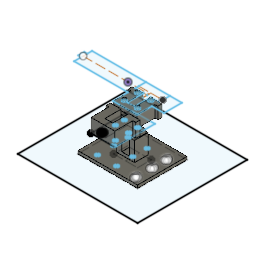
launcher v22 (Autodesk Fusion 360 design; units mm, degrees)
Autodesk Fusion 360 part; units mm, degrees
sketch "草图5" plane through (0, 0, 0) normal (0, 0, 1) x (1, 0, 0)
  line L0 (75, 15) -> (75, -15)
  line L1 (75, 15) -> (-75, 15)
  line L2 (-75, 0) -> (35, 0) construction
  line L3 (35, 3) -> (35, -3) construction
  line L4 (15, 3) -> (55, 3) construction
  line L5 (15, 3) -> (15, -3)
  line L6 (55, -3) -> (55, 3)
  line L7 (55.0002, -15) -> (55.0002, -40)
  line L8 (55.0002, -40) -> (15, -40)
  line L9 (15, -40) -> (15, -15)
  line L10 (35, -3) -> (35.0001, -3)
  line L11 (35.0001, -3) -> (35.0001, -10) construction
  line L12 (35.0001, -10) -> (35, -10)
  line L13 (35, -10) -> (35, -3) construction
  line L14 (29.0001, -3) -> (29.0001, -30)
  line L15 (40.9999, -3) -> (40.9999, -30)
  line L16 (29.0001, -30) -> (40.9999, -30)
  line L17 (55.0002, -15) -> (75, -15)
  line L18 (-75, -15) -> (15, -15)
  line L19 (35, -10) -> (35.0001, -10) construction
  line L20 (29.0001, -3) -> (35.0001, -3) construction
  line L21 (40.9999, -3) -> (42.0001, -3) construction
  line L22 (40.9999, -3) -> (55, -3)
  line L23 (15, -3) -> (29.0001, -3)
  line L24 (35, -3) -> (35.0001, -3)
  line L25 (25, -7) -> (25, -5)
  line L26 (27, -7) -> (27, -9)
  line L27 (23, -5) -> (23, -7)
  line L28 (23, -11) -> (23, -9)
  line L29 (25, -7) -> (27, -7)
  line L30 (25, -9) -> (25, -11)
  line L31 (21, -9) -> (23, -9)
  line L32 (25, -9) -> (25, -7) construction
  line L33 (25, -7) -> (25, -9) construction
  line L34 (25, -9) -> (23, -9) construction
  line L35 (23, -7) -> (21, -7)
  line L36 (23, -9) -> (23, -7) construction
  line L37 (23, -7) -> (25, -7) construction
  line L38 (23, -9) -> (25, -9) construction
  line L39 (21, -7) -> (21, -9)
  line L40 (23, -7) -> (25, -7) construction
  line L41 (27, -9) -> (25, -9)
  line L42 (25, -11) -> (23, -11)
  line L43 (23, -9) -> (23, -7) construction
  line L44 (25, -5) -> (23, -5)
  line L45 (47, -11) -> (47, -9)
  line L46 (47, -9) -> (47, -7) construction
  line L47 (45, -9) -> (47, -9) construction
  line L48 (47, -7) -> (49, -7)
  line L49 (45, -7) -> (45, -9) construction
  line L50 (43, -9) -> (45, -9)
  line L51 (47, -5) -> (47, -7)
  line L52 (45, -11) -> (47, -11)
  line L53 (49, -9) -> (47, -9)
  line L54 (47, -9) -> (45, -9) construction
  line L55 (45, -5) -> (47, -5)
  line L56 (47, -7) -> (45, -7) construction
  line L57 (45, -9) -> (45, -11)
  line L58 (45, -7) -> (43, -7)
  line L59 (47, -9) -> (47, -7) construction
  line L60 (45, -9) -> (45, -7) construction
  line L61 (45, -7) -> (45, -5)
  line L62 (49, -7) -> (49, -9)
  line L63 (43, -7) -> (43, -9)
  line L64 (47, -7) -> (45, -7) construction
  line L65 (25, -31) -> (25, -29) construction
  line L66 (27, -29) -> (27, -31)
  line L67 (25, -29) -> (27, -29)
  line L68 (23, -31) -> (23, -29) construction
  line L69 (25, -29) -> (25, -31) construction
  line L70 (25, -31) -> (25, -33)
  line L71 (21, -31) -> (23, -31)
  line L72 (23, -29) -> (25, -29) construction
  line L73 (25, -33) -> (23, -33)
  line L74 (21, -29) -> (21, -31)
  line L75 (25, -27) -> (23, -27)
  line L76 (27, -31) -> (25, -31)
  line L77 (25, -31) -> (23, -31) construction
  line L78 (23, -31) -> (25, -31) construction
  line L79 (23, -33) -> (23, -31)
  line L80 (23, -31) -> (23, -29) construction
  line L81 (23, -27) -> (23, -29)
  line L82 (23, -29) -> (25, -29) construction
  line L83 (23, -29) -> (21, -29)
  line L84 (25, -29) -> (25, -27)
  line L85 (47, -31) -> (47, -29) construction
  line L86 (49, -29) -> (49, -31)
  line L87 (43, -29) -> (43, -31)
  line L88 (47, -27) -> (47, -29)
  line L89 (45, -31) -> (45, -29) construction
  line L90 (49, -31) -> (47, -31)
  line L91 (47, -29) -> (49, -29)
  line L92 (47, -29) -> (45, -29) construction
  line L93 (45, -29) -> (45, -31) construction
  line L94 (45, -31) -> (47, -31) construction
  line L95 (45, -29) -> (45, -27)
  line L96 (45, -27) -> (47, -27)
  line L97 (45, -31) -> (45, -33)
  line L98 (47, -33) -> (47, -31)
  line L99 (47, -31) -> (45, -31) construction
  line L100 (47, -31) -> (47, -29) construction
  line L101 (45, -29) -> (43, -29)
  line L102 (47, -29) -> (45, -29) construction
  line L103 (43, -31) -> (45, -31)
  line L104 (45, -33) -> (47, -33)
  line L105 (-75, 7) -> (-75, -3) construction
  line L106 (-75, 7) -> (-80, 7)
  line L107 (-75, -3) -> (-80, -3)
  line L108 (-80, -3) -> (-80, 7)
  line L109 (-75, 15) -> (-75, 7)
  line L110 (-75, -3) -> (-75, -15)
  line L111 (15, 3) -> (15, 15)
  line L112 (55, 3) -> (55, 15)
  point P0 (55, 3)
  dimension "d46" = 30
  dimension "d47" = 110
  dimension "d48" = 150
  dimension "d49" = 6
  dimension "d50" = 40
  dimension "d51" = 13
  dimension "d52" = 27
  dimension "d60" = 2
  dimension "d61" = 2
  dimension "d62" = 2
  dimension "d63" = 2
  dimension "d64" = 2
  dimension "d65" = 2
  dimension "d66" = 2
  dimension "d67" = 2
  dimension "d68" = 2
  dimension "d69" = 2
  dimension "d70" = 2
  dimension "d71" = 2
  dimension "d148" = 10
  dimension "d149" = 5
  constraint vertical L0
  constraint perpendicular L1 L109
  constraint perpendicular L0 L1
  constraint perpendicular L2 L3
  constraint midpoint L2.end L3
  constraint horizontal L4
  constraint midpoint L3.start L4
  constraint symmetric L2 P0 L6.start
  constraint perpendicular L5 L23
  constraint vertical L7
  constraint horizontal L8
  constraint vertical L9
  constraint vertical L11
  constraint horizontal L12
  constraint vertical L13
  constraint coincident L21.end L23
  constraint parallel L20 L23
  constraint perpendicular L14 L23
  constraint symmetric L13 L14.start L15.start
  constraint symmetric L13 L14.end L15.end
  constraint collinear L17 L18
  constraint collinear L20 L21
  constraint collinear L22 L23
  constraint collinear L23 L24
  constraint horizontal L37
  constraint vertical L33
  constraint horizontal L34
  constraint vertical L36
  constraint horizontal L29
  constraint vertical L26
  constraint horizontal L41
  constraint vertical L32
  constraint horizontal L35
  constraint vertical L39
  constraint horizontal L31
  constraint vertical L43
  constraint horizontal L40
  constraint vertical L25
  constraint horizontal L44
  constraint vertical L27
  constraint horizontal L38
  constraint vertical L30
  constraint horizontal L42
  constraint vertical L28
  constraint symmetric L3 L4.start P0
  constraint symmetric L3 L35.end L48.end
  constraint symmetric L3 L31.start L53.start
  constraint symmetric L3 L26.start L58.end
  constraint symmetric L3 L25.start L49.start
  constraint symmetric L3 L27.end L46.end
  constraint symmetric L3 L25.end L55.start
  constraint symmetric L3 L27.start L51.start
  constraint symmetric L3 L30.start L47.start
  constraint symmetric L3 L30.end L52.start
  constraint symmetric L3 L28.start L45.start
  constraint symmetric L3 L28.end L45.end
  constraint symmetric L3 L26.end L50.start
  constraint horizontal L82
  constraint vertical L69
  constraint horizontal L77
  constraint vertical L68
  constraint horizontal L67
  constraint vertical L66
  constraint horizontal L76
  constraint vertical L65
  constraint horizontal L83
  constraint vertical L74
  constraint horizontal L71
  constraint vertical L80
  constraint horizontal L72
  constraint vertical L84
  constraint horizontal L75
  constraint vertical L81
  constraint horizontal L78
  constraint vertical L70
  constraint horizontal L73
  constraint vertical L79
  constraint symmetric L3 L65.start L89.start
  constraint symmetric L3 L68.start L85.start
  constraint symmetric L3 L70.end L97.end
  constraint symmetric L3 L73.end L98.start
  constraint symmetric L3 L66.end L87.end
  constraint symmetric L3 L75.start L95.end
  constraint symmetric L3 L65.end L89.end
  constraint symmetric L3 L75.end L88.start
  constraint symmetric L3 L68.end L85.end
  constraint symmetric L3 L74.start L86.start
  constraint symmetric L3 L66.start L87.start
  constraint symmetric L3 L71.start L86.end
  constraint symmetric L7 L9 L11
  constraint coincident L105.end L109
  constraint perpendicular L106 L109
  constraint perpendicular L105 L107
  constraint equal L106 L107
  constraint collinear L109 L110
  constraint coincident L1 L111.end
  constraint perpendicular L1 L111
  constraint coincident P0 L4.end
  constraint coincident L1 L112.end
  constraint perpendicular L1 L112
  measures "d46" distance of L1.end L18.start
  measures "d47" distance of L2.start L2.end
  measures "d48" distance of L1.end L0.start
  measures "d49" distance of L3.start L3.end
  measures "d50" distance of L4.start P0
  measures "d51" distance of L14.start L21.end
  measures "d52" distance of L14.start L14.end
  measures "d60" distance of L27.end L28.end
  measures "d61" distance of L27.end L25.start
  measures "d62" distance of L26.start L25.start
  measures "d63" distance of L35.end L27.end
  measures "d64" distance of L27.end L27.start
  measures "d65" distance of L28.start L28.end
  measures "d66" distance of L68.start L68.end
  measures "d67" distance of L65.end L68.end
  measures "d68" distance of L65.end L66.start
  measures "d69" distance of L68.end L74.start
  measures "d70" distance of L75.end L68.end
  measures "d71" distance of L68.start L73.end
  measures "d148" distance of L105.start L105.end
  measures "d149" distance of L105.start L106.end
sketch "草图8" plane through (0, 0, 0) normal (0, 0, 1) x (1, 0, 0)
  line L0 (49, -31) -> (47, -31)
  line L1 (43, -29) -> (43, -31)
  line L2 (45, -29) -> (43, -29)
  line L3 (45, -29) -> (45, -31) construction
  line L4 (28.5, -3) -> (28.5, -30)
  line L5 (35, -10) -> (35, -3) construction
  line L6 (27, -31) -> (25, -31)
  line L7 (27, -29) -> (27, -31)
  line L8 (23, -27) -> (23, -29)
  line L9 (25, -29) -> (27, -29)
  line L10 (41.5, -3) -> (41.5, -30)
  line L11 (43, -31) -> (45, -31)
  line L12 (25, -31) -> (25, -29) construction
  line L13 (35, -3) -> (35.0001, -3)
  line L14 (45, -33) -> (47, -33)
  line L15 (47, -31) -> (47, -29) construction
  line L16 (23, -31) -> (25, -31) construction
  line L17 (25, -33) -> (23, -33)
  line L18 (55, -10) -> (55, -40)
  line L19 (41.5, -3) -> (51, -3)
  line L20 (47, -29) -> (45, -29) construction
  line L21 (47, -29) -> (45, -29) construction
  line L22 (47, -27) -> (47, -29)
  line L23 (47, -31) -> (45, -31) construction
  line L24 (45, -27) -> (47, -27)
  line L25 (49, -29) -> (49, -31)
  line L26 (23, -31) -> (23, -29) construction
  line L27 (25, -31) -> (25, -33)
  line L28 (35, -10) -> (35.0001, -10) construction
  line L29 (35.0001, -3) -> (35.0001, -10) construction
  line L30 (35.0001, -10) -> (35, -10)
  line L31 (23, -31) -> (23, -29) construction
  line L32 (28.5, -3) -> (35.0001, -3) construction
  line L33 (23, -33) -> (23, -31)
  line L34 (23, -29) -> (25, -29) construction
  line L35 (45, -5) -> (47, -5)
  line L36 (47, -7) -> (45, -7) construction
  line L37 (45, -9) -> (45, -7) construction
  line L38 (47, -7) -> (49, -7)
  line L39 (21, -31) -> (23, -31)
  line L40 (23, -29) -> (21, -29)
  line L41 (47, -11) -> (47, -9)
  line L42 (47, -5) -> (47, -7)
  line L43 (49, -7) -> (49, -9)
  line L44 (19, -3) -> (28.5, -3)
  line L45 (45, -7) -> (45, -9) construction
  line L46 (55, -40) -> (15, -40)
  line L47 (49, -9) -> (47, -9)
  line L48 (23, -7) -> (21, -7)
  line L49 (47, -7) -> (45, -7) construction
  line L50 (28.5, -30) -> (41.5, -30)
  line L51 (45, -11) -> (47, -11)
  line L52 (21, -29) -> (21, -31)
  line L53 (25, -7) -> (25, -5)
  line L54 (45, -7) -> (43, -7)
  line L55 (43, -7) -> (43, -9)
  line L56 (15, -40) -> (15, -10)
  line L57 (47, -33) -> (47, -31)
  line L58 (45, -29) -> (45, -27)
  line L59 (45, -31) -> (45, -29) construction
  line L60 (47, -29) -> (49, -29)
  line L61 (23, -29) -> (25, -29) construction
  line L62 (25, -27) -> (23, -27)
  line L63 (25, -29) -> (25, -27)
  line L64 (25, -29) -> (25, -31) construction
  line L65 (25, -31) -> (23, -31) construction
  line L66 (35, -3) -> (35.0001, -3)
  line L67 (25, -7) -> (27, -7)
  line L68 (23, -7) -> (25, -7) construction
  line L69 (27, -7) -> (27, -9)
  line L70 (25, -7) -> (25, -9) construction
  line L71 (47, -9) -> (47, -7) construction
  line L72 (45, -9) -> (47, -9) construction
  line L73 (27, -9) -> (25, -9)
  line L74 (23, -5) -> (23, -7)
  line L75 (25, -5) -> (23, -5)
  line L76 (23, -9) -> (23, -7) construction
  line L77 (21, -9) -> (23, -9)
  line L78 (25, -9) -> (25, -11)
  line L79 (23, -9) -> (25, -9) construction
  line L80 (25, -9) -> (25, -7) construction
  line L81 (25, -11) -> (23, -11)
  line L82 (25, -9) -> (23, -9) construction
  line L83 (47, -9) -> (47, -7) construction
  line L84 (23, -7) -> (25, -7) construction
  line L85 (21, -7) -> (21, -9)
  line L86 (43, -9) -> (45, -9)
  line L87 (47, -9) -> (45, -9) construction
  line L88 (23, -9) -> (23, -7) construction
  line L89 (45, -9) -> (45, -11)
  line L90 (23, -11) -> (23, -9)
  line L91 (45, -31) -> (47, -31) construction
  line L92 (45, -31) -> (45, -33)
  line L93 (41.5, -3) -> (42.0001, -3) construction
  line L94 (47, -31) -> (47, -29) construction
  line L95 (45, -7) -> (45, -5)
  line L96 (15, -10) -> (10, -10)
  line L97 (55, -10) -> (60, -10)
  line L98 (28.5, -13.5) -> (41.5, -13.5)
  line L99 (28.5, -10.5) -> (41.5, -10.5)
  line L100 (35, -10) -> (35, -30) construction
  line L101 (10, -3) -> (60, -3)
  line L102 (10, -3) -> (10, -10)
  line L103 (60, -3) -> (60, -10)
  point P0 (35, 0)
  point P1 (51, 3)
  dimension "d90" = 27
  dimension "d91" = 2
  dimension "d92" = 2
  dimension "d93" = 2
  dimension "d94" = 2
  dimension "d95" = 2
  dimension "d96" = 2
  dimension "d97" = 2
  dimension "d98" = 2
  dimension "d99" = 2
  dimension "d100" = 2
  dimension "d101" = 2
  dimension "d102" = 2
  dimension "d105" = 16.5
  dimension "d106" = 3
  dimension "d134" = 13
  constraint vertical L18
  constraint horizontal L46
  constraint vertical L56
  constraint vertical L29
  constraint horizontal L30
  constraint vertical L5
  constraint coincident L93.end L44
  constraint parallel L32 L44
  constraint perpendicular L4 L44
  constraint symmetric L4.start L10.start L5
  constraint symmetric L10.end L4.end L5
  constraint collinear L32 L93
  constraint collinear L19 L44
  constraint collinear L13 L44
  constraint horizontal L84
  constraint vertical L70
  constraint horizontal L82
  constraint vertical L88
  constraint horizontal L67
  constraint vertical L69
  constraint horizontal L73
  constraint vertical L80
  constraint horizontal L48
  constraint vertical L85
  constraint horizontal L77
  constraint vertical L76
  constraint horizontal L68
  constraint vertical L53
  constraint horizontal L75
  constraint vertical L74
  constraint horizontal L79
  constraint vertical L78
  constraint horizontal L81
  constraint vertical L90
  constraint horizontal L61
  constraint vertical L64
  constraint horizontal L65
  constraint vertical L31
  constraint horizontal L9
  constraint vertical L7
  constraint horizontal L6
  constraint vertical L12
  constraint horizontal L40
  constraint vertical L52
  constraint horizontal L39
  constraint vertical L26
  constraint horizontal L34
  constraint vertical L63
  constraint horizontal L62
  constraint vertical L8
  constraint horizontal L16
  constraint vertical L27
  constraint horizontal L17
  constraint vertical L33
  constraint perpendicular L56 L96
  constraint coincident L4 L98.start
  constraint coincident L10 L98.end
  constraint perpendicular L10 L98
  constraint coincident L4 L99.start
  constraint coincident L10 L99.end
  constraint perpendicular L10 L99
  constraint midpoint L50 L100.end
  constraint perpendicular L96 L102
  constraint perpendicular L97 L103
  measures "d90" distance of L4.start L4.end
  measures "d91" distance of L76.start L48.start
  measures "d92" distance of L53.start L48.start
  measures "d93" distance of L53.start L67.end
  measures "d94" distance of L48.start L48.end
  measures "d95" distance of L74.start L48.start
  measures "d96" distance of L76.start L81.end
  measures "d97" distance of L8.end L16.start
  measures "d98" distance of L8.end L9.start
  measures "d99" distance of L9.start L7.start
  measures "d100" distance of L40.end L8.end
  measures "d101" distance of L8.start L8.end
  measures "d102" distance of L17.end L16.start
  measures "d105" distance of L50 L98
  measures "d106" distance of L98 L99
  measures "d134" distance of L10.end L4.end
extrude "拉伸10" add sketch "草图8" along normal blind 3 contours L0 L1 L2 L11 L14 L22 L24 L25 L57 L58 L60 L92 | L6 L7 L8 L9 L17 L27 L33 L39 L40 L52 L62 L63 | L35 L38 L41 L42 L43 L47 L51 L54 L55 L86 L89 L95 | L48 L53 L67 L69 L73 L74 L75 L77 L78 L81 L85 L90 makes body 1 at (44.3333, -8.3333, 0) makes body 2 at (46.3333, -31.6667, 0) makes body 3 at (24.3333, -9.6667, 0) makes body 4 at (22.3333, -30.3333, 0)
extrude "拉伸11" add sketch "草图8" against normal blind 20 contours L0 L1 L2 L11 L14 L22 L24 L25 L57 L58 L60 L92 | L4 L10 L99 L101 | L4 L10 L18 L19 L44 L46 L50 L56 L96 L97 L101 L102 L103 | L4 L10 L98 L99 | L4 L10 L50 L98 | L6 L7 L8 L9 L17 L27 L33 L39 L40 L52 L62 L63 | L35 L38 L41 L42 L43 L47 L51 L54 L55 L86 L89 L95 | L48 L53 L67 L69 L73 L74 L75 L77 L78 L81 L85 L90 bodies 1 2 3 4
extrude "拉伸12" cut sketch "草图8" against normal blind 17 contours L4 L10 L98 L99 | L4 L10 L50 L98 bodies 1
extrude "拉伸13" cut sketch "草图8" against normal blind 20 contours L4 L10 L98 L99 bodies 1
extrude "拉伸19" cut sketch "草图8" against normal blind 20 contours L0 L1 L2 L11 L14 L22 L24 L25 L57 L58 L60 L92 | L4 L10 L99 L101 | L4 L10 L18 L19 L44 L46 L50 L56 L96 L97 L101 L102 L103 | L4 L10 L98 L99 | L4 L10 L50 L98 | L6 L7 L8 L9 L17 L27 L33 L39 L40 L52 L62 L63 | L35 L38 L41 L42 L43 L47 L51 L54 L55 L86 L89 L95 | L48 L53 L67 L69 L73 L74 L75 L77 L78 L81 L85 L90 bodies 1 makes body 5 at (22.3333, -30.3333, 0) makes body 6 at (24.3333, -9.6667, 3) makes body 7 at (46.3333, -31.6667, 0)
sketch "草图11" plane through (0, 0, 0) normal (0, 0, 1) x (1, 0, 0)
  line L0 (15, -35, -5) -> (55, -35, -5)
  line L1 (55, -35, -5) -> (55, -35, -15)
  line L2 (55, -35, -15) -> (15, -35, -15)
  line L3 (15, -35, -15) -> (15, -35, -5)
  circle A0 through (38.5, -35, -10) (33.25, -35, -6.9689) (33.25, -35, -13.0311)
  circle A1 through (38, -35, -10) (33.5, -35, -7.4019) (33.5, -35, -12.5981) construction
  line L4 (35, -35, -5) -> (35, -35, -15) construction
  line L5 (35, -35, -10) -> (49, -35, -10) construction
  circle A2 through (51, -35, -10) (48, -35, -8.2679) (48, -35, -11.7321)
  line L6 (35, -35, -6.9923) -> (49.1429, -35, -8.0051)
  line L7 (35, -35, -13.0077) -> (49.1429, -35, -11.9949)
  line L8 (35, -35, -6.9923) -> (20.8571, -35, -8.0051)
  line L9 (35, -35, -13.0077) -> (20.8571, -35, -11.9949)
  line L10 (35, -35, -10) -> (21, -35, -10) construction
  circle A3 through (23, -35, -10) (20, -35, -8.2679) (20, -35, -11.7321)
  dimension "d141" = 7
  dimension "d142" = 6
  dimension "d143" = 4
  dimension "d154" = 14
extrude "拉伸21" add sketch "草图8" against normal blind 20 contours L0 L1 L2 L11 L14 L22 L24 L25 L57 L58 L60 L92 | L4 L10 L99 L101 | L4 L10 L18 L19 L44 L46 L50 L56 L96 L97 L101 L102 L103 | L4 L10 L50 L98 | L6 L7 L8 L9 L17 L27 L33 L39 L40 L52 L62 L63 | L35 L38 L41 L42 L43 L47 L51 L54 L55 L86 L89 L95 | L48 L53 L67 L69 L73 L74 L75 L77 L78 L81 L85 L90 bodies 1 5 6 7
extrude "拉伸22" cut sketch "草图8" against normal blind 17 contours L4 L10 L99 L101 | L4 L10 L50 L98 bodies 1
extrude "拉伸23" cut sketch "草图11" against normal blind 6 contours A0 L6 L7 L8 L9 | A0 L8 L9 A3 | A0 L6 L8 | A0 L7 L9 | A0 A2 L6 L7 | A3 | A2 in plane through (0, -35, 0) normal (0, 1, 0) bodies 1
copy_body "复制和粘贴实体1" bodies 1 makes body 8
move_body "移动1" bodies 8 to x (1, 0, 0) y (0, 1, 0) z (0, 0, 1) at (-72, -41, 20)
extrude "拉伸24" add 1 faces at (-43.0559, -76, 9.335) along direction (0, -1, 0) blind 5 on bodies 8 bodies 8
extrude "拉伸25" add 4 faces at (-27.6667, -49.3333, 23) (-49.6667, -48.6667, 23) (-49.6667, -71.3333, 23) (-25.6667, -72.6667, 23) along direction (0, 0, -1) blind 28 on bodies 8 bodies 8
extrude "拉伸26" cut 4 faces at (-49.6667, -48.6667, 23) (-27.6667, -49.3333, 23) (-25.6667, -72.6667, 23) (-49.6667, -71.3333, 23) along direction (0, 0, -1) blind 3 on bodies 8 bodies 8
extrude "拉伸27" add 1 faces at (-39.1667, -64.8333, 0) along direction (0, 0, -1) blind 2 on bodies 8 bodies 8
extrude "拉伸28" add 1 faces at (-39.1667, -64.8333, -2) along direction (0, 0, -1) blind 1 on bodies 8 bodies 8
extrude "拉伸29" add 4 faces at (-27.6667, -49.3333, -5) (-49.6667, -48.6667, -5) (-49.6667, -71.3333, -5) (-25.6667, -72.6667, -5) along direction (0, 0, -1) blind 1 on bodies 8 bodies 8
move_body "移动2" bodies 8 to x (1, 0, 0) y (0, 1, 0) z (0, 0, 1) at (72, 4, -25)
sketch "草图12" plane through (0, 0, -28) normal (0, 0, -1) x (1, 0, 0)
  line L0 (43, 66) -> (43, 68)
  line L1 (43, 68) -> (45, 68)
  line L2 (45, 68) -> (45, 70)
  line L3 (45, 70) -> (47, 70)
  line L4 (47, 70) -> (47, 68)
  line L5 (47, 68) -> (49, 68)
  line L6 (49, 68) -> (49, 66)
  line L7 (49, 66) -> (47, 66)
  line L8 (47, 66) -> (47, 64)
  line L9 (47, 64) -> (45, 64)
  line L10 (45, 64) -> (45, 66)
  line L11 (45, 66) -> (43, 66)
  line L12 (25, 42) -> (23, 42)
  line L13 (23, 42) -> (23, 44)
  line L14 (23, 44) -> (21, 44)
  line L15 (21, 44) -> (21, 46)
  line L16 (21, 46) -> (23, 46)
  line L17 (23, 46) -> (23, 48)
  line L18 (23, 48) -> (25, 48)
  line L19 (25, 48) -> (25, 46)
  line L20 (25, 46) -> (27, 46)
  line L21 (27, 46) -> (27, 44)
  line L22 (27, 44) -> (25, 44)
  line L23 (25, 44) -> (25, 42)
  line L24 (43, 46) -> (45, 46)
  line L25 (45, 46) -> (45, 48)
  line L26 (45, 48) -> (47, 48)
  line L27 (47, 48) -> (47, 46)
  line L28 (47, 46) -> (49, 46)
  line L29 (49, 46) -> (49, 44)
  line L30 (49, 44) -> (47, 44)
  line L31 (47, 44) -> (47, 42)
  line L32 (47, 42) -> (45, 42)
  line L33 (45, 42) -> (45, 44)
  line L34 (45, 44) -> (43, 44)
  line L35 (43, 44) -> (43, 46)
  line L36 (25, 66) -> (25, 64)
  line L37 (25, 64) -> (23, 64)
  line L38 (23, 64) -> (23, 66)
  line L39 (23, 66) -> (21, 66)
  line L40 (21, 66) -> (21, 68)
  line L41 (21, 68) -> (23, 68)
  line L42 (23, 68) -> (23, 70)
  line L43 (23, 70) -> (25, 70)
  line L44 (25, 70) -> (25, 68)
  line L45 (25, 68) -> (27, 68)
  line L46 (27, 68) -> (27, 66)
  line L47 (27, 66) -> (25, 66)
  line L48 (28.5, 50.5) -> (41.5, 50.5)
  line L49 (41.5, 50.5) -> (41.5, 47.5)
  line L50 (41.5, 47.5) -> (28.5, 47.5)
  line L51 (28.5, 47.5) -> (28.5, 50.5)
  line L52 (10, 47) -> (10, 40)
  line L53 (10, 40) -> (60, 40)
  line L54 (60, 40) -> (60, 47)
  line L55 (60, 47) -> (55, 47)
  line L56 (55, 47) -> (55, 77)
  line L57 (55, 77) -> (15, 77)
  line L58 (15, 77) -> (15, 47)
  line L59 (15, 47) -> (10, 47)
  line L60 (15, 77) -> (55, 77)
  line L61 (55, 77) -> (55, 10)
  line L62 (55, 10) -> (15, 10)
  line L63 (15, 10) -> (15, 77)
  line L64 (21, 68) -> (23, 68)
  line L65 (23, 70) -> (25, 70)
  line L66 (25, 68) -> (27, 68)
  line L67 (27, 66) -> (25, 66)
  line L68 (25, 64) -> (23, 64)
  line L69 (23, 66) -> (21, 66)
  line L70 (25, 70) -> (25, 68)
  line L71 (27, 68) -> (27, 66)
  line L72 (25, 66) -> (25, 64)
  line L73 (23, 64) -> (23, 66)
  line L74 (21, 66) -> (21, 68)
  line L75 (23, 68) -> (23, 70)
  line L76 (47, 66) -> (47, 64)
  line L77 (49, 66) -> (47, 66)
  line L78 (45, 66) -> (43, 66)
  line L79 (43, 68) -> (45, 68)
  line L80 (43, 66) -> (43, 68)
  line L81 (45, 64) -> (45, 66)
  line L82 (47, 64) -> (45, 64)
  line L83 (47, 70) -> (47, 68)
  line L84 (47, 64) -> (45, 64)
  line L85 (47, 70) -> (47, 68)
  line L86 (49, 68) -> (49, 66)
  line L87 (47, 68) -> (49, 68)
  line L88 (45, 68) -> (45, 70)
  line L89 (43, 66) -> (43, 68)
  line L90 (47, 66) -> (47, 64)
  line L91 (45, 64) -> (45, 66)
  line L92 (43, 68) -> (45, 68)
  line L93 (49, 66) -> (47, 66)
  line L94 (45, 70) -> (47, 70)
  line L95 (47, 68) -> (49, 68)
  line L96 (45, 68) -> (45, 70)
  line L97 (45, 66) -> (43, 66)
  line L98 (45, 70) -> (47, 70)
  line L99 (49, 68) -> (49, 66)
  line L100 (47, 46) -> (49, 46)
  line L101 (49, 46) -> (49, 44)
  line L102 (49, 44) -> (47, 44)
  line L103 (47, 44) -> (47, 42)
  line L104 (25, 46) -> (27, 46)
  line L105 (45, 42) -> (45, 44)
  line L106 (27, 46) -> (27, 44)
  line L107 (25, 46) -> (27, 46)
  line L108 (23, 48) -> (25, 48)
  line L109 (45, 44) -> (43, 44)
  line L110 (27, 44) -> (25, 44)
  line L111 (45, 48) -> (47, 48)
  line L112 (45, 46) -> (45, 48)
  line L113 (47, 44) -> (47, 42)
  line L114 (47, 44) -> (47, 42)
  line L115 (21, 46) -> (23, 46)
  line L116 (49, 44) -> (47, 44)
  line L117 (25, 48) -> (25, 46)
  line L118 (49, 46) -> (49, 44)
  line L119 (45, 42) -> (45, 44)
  line L120 (25, 44) -> (25, 42)
  line L121 (21, 44) -> (21, 46)
  line L122 (23, 46) -> (23, 48)
  line L123 (27, 46) -> (27, 44)
  line L124 (23, 42) -> (23, 44)
  line L125 (21, 46) -> (23, 46)
  line L126 (49, 44) -> (47, 44)
  line L127 (25, 42) -> (23, 42)
  line L128 (23, 44) -> (21, 44)
  line L129 (23, 48) -> (25, 48)
  line L130 (23, 42) -> (23, 44)
  line L131 (23, 46) -> (23, 48)
  line L132 (25, 42) -> (23, 42)
  line L133 (23, 44) -> (21, 44)
  line L134 (25, 44) -> (25, 42)
  line L135 (47, 42) -> (45, 42)
  line L136 (45, 46) -> (45, 48)
  line L137 (47, 48) -> (47, 46)
  line L138 (25, 48) -> (25, 46)
  line L139 (21, 44) -> (21, 46)
  line L140 (45, 48) -> (47, 48)
  line L141 (43, 46) -> (45, 46)
  line L142 (49, 46) -> (49, 44)
  line L143 (27, 44) -> (25, 44)
  line L144 (43, 44) -> (43, 46)
  line L145 (47, 48) -> (47, 46)
  line L146 (47, 46) -> (49, 46)
  line L147 (47, 48) -> (47, 46)
  line L148 (45, 46) -> (45, 48)
  line L149 (45, 48) -> (47, 48)
  line L150 (47, 46) -> (49, 46)
  line L151 (47, 42) -> (45, 42)
  line L152 (45, 44) -> (43, 44)
  line L153 (43, 46) -> (45, 46)
  line L154 (43, 44) -> (43, 46)
  line L155 (43, 44) -> (43, 46)
  line L156 (45, 42) -> (45, 44)
  line L157 (45, 44) -> (43, 44)
  line L158 (47, 42) -> (45, 42)
  line L159 (43, 46) -> (45, 46)
  line L160 (47, 31) -> (49, 31)
  line L161 (49, 31) -> (49, 29)
  line L162 (49, 29) -> (47, 29)
  line L163 (47, 29) -> (47, 27)
  line L164 (25, 31) -> (27, 31)
  line L165 (45, 27) -> (45, 29)
  line L166 (27, 31) -> (27, 29)
  line L167 (25, 31) -> (27, 31)
  line L168 (23, 33) -> (25, 33)
  line L169 (45, 29) -> (43, 29)
  line L170 (27, 29) -> (25, 29)
  line L171 (45, 33) -> (47, 33)
  line L172 (45, 31) -> (45, 33)
  line L173 (47, 29) -> (47, 27)
  line L174 (47, 29) -> (47, 27)
  line L175 (21, 31) -> (23, 31)
  line L176 (49, 29) -> (47, 29)
  line L177 (25, 33) -> (25, 31)
  line L178 (49, 31) -> (49, 29)
  line L179 (45, 27) -> (45, 29)
  line L180 (25, 29) -> (25, 27)
  line L181 (21, 29) -> (21, 31)
  line L182 (23, 31) -> (23, 33)
  line L183 (27, 31) -> (27, 29)
  line L184 (23, 27) -> (23, 29)
  line L185 (21, 31) -> (23, 31)
  line L186 (49, 29) -> (47, 29)
  line L187 (25, 27) -> (23, 27)
  line L188 (23, 29) -> (21, 29)
  line L189 (23, 33) -> (25, 33)
  line L190 (23, 27) -> (23, 29)
  line L191 (23, 31) -> (23, 33)
  line L192 (25, 27) -> (23, 27)
  line L193 (23, 29) -> (21, 29)
  line L194 (25, 29) -> (25, 27)
  line L195 (47, 27) -> (45, 27)
  line L196 (45, 31) -> (45, 33)
  line L197 (47, 33) -> (47, 31)
  line L198 (25, 33) -> (25, 31)
  line L199 (21, 29) -> (21, 31)
  line L200 (45, 33) -> (47, 33)
  line L201 (43, 31) -> (45, 31)
  line L202 (49, 31) -> (49, 29)
  line L203 (27, 29) -> (25, 29)
  line L204 (43, 29) -> (43, 31)
  line L205 (47, 33) -> (47, 31)
  line L206 (47, 31) -> (49, 31)
  line L207 (47, 33) -> (47, 31)
  line L208 (45, 31) -> (45, 33)
  line L209 (45, 33) -> (47, 33)
  line L210 (47, 31) -> (49, 31)
  line L211 (47, 27) -> (45, 27)
  line L212 (45, 29) -> (43, 29)
  line L213 (43, 31) -> (45, 31)
  line L214 (43, 29) -> (43, 31)
  line L215 (43, 29) -> (43, 31)
  line L216 (45, 27) -> (45, 29)
  line L217 (45, 29) -> (43, 29)
  line L218 (47, 27) -> (45, 27)
  line L219 (43, 31) -> (45, 31)
  constraint horizontal L60
  constraint vertical L61
  constraint horizontal L62
  constraint vertical L63
  constraint coincident L57.end L58.start
  constraint coincident L40.end L41.start
  constraint coincident L41.end L42.start
  constraint coincident L42.end L43.start
  constraint coincident L43.end L44.start
  constraint coincident L44.end L45.start
  constraint coincident L45.end L46.start
  constraint coincident L46.end L47.start
  constraint coincident L36.start L47.end
  constraint coincident L36.end L37.start
  constraint coincident L37.end L38.start
  constraint coincident L38.end L39.start
  constraint coincident L39.end L40.start
  constraint coincident L0.end L1.start
  constraint coincident L1.end L2.start
  constraint coincident L2.end L3.start
  constraint coincident L3.end L4.start
  constraint coincident L4.end L5.start
  constraint coincident L5.end L6.start
  constraint coincident L6.end L7.start
  constraint coincident L7.end L8.start
  constraint coincident L8.end L9.start
  constraint coincident L9.end L10.start
  constraint coincident L10.end L11.start
  constraint coincident L0.start L11.end
  constraint coincident L15.end L16.start
  constraint coincident L16.end L17.start
  constraint coincident L17.end L18.start
  constraint coincident L18.end L19.start
  constraint coincident L19.end L20.start
  constraint coincident L20.end L21.start
  constraint coincident L21.end L22.start
  constraint coincident L22.end L23.start
  constraint coincident L12.start L23.end
  constraint coincident L12.end L13.start
  constraint coincident L13.end L14.start
  constraint coincident L14.end L15.start
  constraint coincident L24.start L35.end
  constraint coincident L24.end L25.start
  constraint coincident L25.end L26.start
  constraint coincident L26.end L27.start
  constraint coincident L27.end L28.start
  constraint coincident L28.end L29.start
  constraint coincident L29.end L30.start
  constraint coincident L30.end L31.start
  constraint coincident L31.end L32.start
  constraint coincident L32.end L33.start
  constraint coincident L33.end L34.start
  constraint coincident L34.end L35.start
  constraint coincident L175.start L181.end
  constraint coincident L175.end L182.start
  constraint coincident L168.start L182.end
  constraint coincident L168.end L177.start
  constraint coincident L164.start L167.start
  constraint coincident L164.end L166.start
  constraint coincident L166.end L170.start
  constraint coincident L170.end L180.start
  constraint coincident L180.end L187.start
  constraint coincident L184.start L187.end
  constraint coincident L184.end L188.start
  constraint coincident L181.start L188.end
  constraint coincident L201.start L204.end
  constraint coincident L172.start L196.start
  constraint coincident L171.start L172.end
  constraint coincident L171.end L197.start
  constraint coincident L160.start L197.end
  constraint coincident L160.end L161.start
  constraint coincident L161.end L162.start
  constraint coincident L162.end L163.start
  constraint coincident L163.end L173.end
  constraint coincident L165.start L179.start
  constraint coincident L165.end L169.start
  constraint coincident L169.end L204.start
sketch "草图13" plane through (0, 0, 0) normal (0, 1, 0) x (1, 0, 0)
  circle A0 through (19, 31, -30) (22, 31, -28.2679) (22, 31, -31.7321)
  line L0 (35, 31, -30) -> (21, 31, -30) construction
  line L1 (35, 31, -30) -> (49, 31, -30) construction
  line L2 (35, 31, -35) -> (35, 31, -25) construction
  line L3 (35, 31, -26.9923) -> (20.8571, 31, -28.0051)
  line L4 (35, 31, -33.0077) -> (20.8571, 31, -31.9949)
  line L5 (35, 31, -26.9923) -> (49.1429, 31, -28.0051)
  circle A1 through (32, 31, -30) (36.5, 31, -27.4019) (36.5, 31, -32.5981) construction
  circle A2 through (31.5, 31, -30) (36.75, 31, -26.9689) (36.75, 31, -33.0311)
  line L6 (35, 31, -33.0077) -> (49.1429, 31, -31.9949)
  line L7 (15, 31, -25) -> (15, 31, -35)
  line L8 (15, 31, -35) -> (55, 31, -35)
  line L9 (55, 31, -35) -> (55, 31, -25)
  circle A3 through (47, 31, -30) (50, 31, -28.2679) (50, 31, -31.7321)
  line L10 (55, 31, -25) -> (15, 31, -25)
  dimension "d183" = 7
  dimension "d184" = 6
  dimension "d185" = 4
  dimension "d186" = 14
extrude "拉伸35" add sketch "草图13" along normal blind 5 separate body contours A0 | A0 L3 L4 A2 | L3 L4 L5 A2 L6 | L3 L5 A2 | L4 A2 L6 | L5 A2 L6 A3 | A3 | L7 L8 L9 L10 in plane through (0, 0, -31) normal (0, 0, -1) makes body 9
extrude "拉伸36" add sketch "草图12" along normal blind 3 contours L160 L161 L162 L163 L165 L169 L171 L172 L173 L174 L176 L178 L179 L186 L195 L196 L197 L200 L201 L202 L204 L205 L206 L207 L208 L209 L210 L211 L212 L213 L214 L215 L216 L217 L218 L219 | L164 L166 L167 L168 L170 L175 L177 L180 L181 L182 L183 L184 L185 L187 L188 L189 L190 L191 L192 L193 L194 L198 L199 L203 bodies 9
extrude "拉伸37" add sketch "草图13" along normal blind 8 contours L7 L8 L9 L10 in plane through (0, 0, -31) normal (0, 0, -1) bodies 9
extrude "拉伸38" cut 1 faces at (41.0559, -29.335, -36) along direction (0, 0, 1) blind 2 on bodies 9 bodies 9
extrude "拉伸39" cut 1 faces at (16.3333, -30, -39) along direction (0, 0, 1) blind 2 on bodies 9 bodies 9
copy_body "复制和粘贴实体2" bodies 8 makes body 10
move_body "移动3" bodies 10 to x (1, 0, 0) y (0, 0, 1) z (0, -1, 0) at (0, -44, 0)
extrude "拉伸40" cut 4 faces at (22.3333, -13, -44.6667) (44.3333, -13, -45.3333) (22.3333, -13, -67.3333) (46.3333, -13, -68.6667) along direction (0, -1, 0) blind 3 on bodies 10 bodies 10
sketch "草图14" plane through (0, 0, -77) normal (0, 0, -1) x (1, 0, 0)
  line L0 (55, 39) -> (15, 39)
  line L1 (15, 39) -> (15, 16)
  line L2 (15, 16) -> (55, 16)
  line L3 (55, 16) -> (55, 39)
  line L4 (2, 57) -> (4, 57)
  line L5 (4, 57) -> (4, 55)
  line L6 (0, 55) -> (2, 55)
  line L7 (4, 57) -> (4, 55)
  line L8 (2, 55) -> (2, 57)
  line L9 (4, 55) -> (6, 55)
  line L10 (0, 55) -> (2, 55)
  line L11 (4, 55) -> (6, 55)
  line L12 (2, 57) -> (4, 57)
  line L13 (2, 55) -> (2, 57)
  line L14 (2, 53) -> (0, 53)
  line L15 (4, 53) -> (4, 51)
  line L16 (2, 53) -> (0, 53)
  line L17 (4, 51) -> (2, 51)
  line L18 (2, 51) -> (2, 53)
  line L19 (4, 51) -> (2, 51)
  line L20 (4, 53) -> (4, 51)
  line L21 (0, 53) -> (0, 55)
  line L22 (6, 55) -> (6, 53)
  line L23 (6, 55) -> (6, 53)
  line L24 (6, 53) -> (4, 53)
  line L25 (0, 53) -> (0, 55)
  line L26 (2, 51) -> (2, 53)
  line L27 (6, 53) -> (4, 53)
  line L28 (15, 39) -> (55, 39)
  line L29 (55, 39) -> (55, 16)
  line L30 (55, 16) -> (15, 16)
  line L31 (15, 16) -> (15, 39)
  line L32 (85, -14) -> (-15, -14)
  line L33 (-15, -14) -> (-15, 69)
  line L34 (-15, 69) -> (85, 69)
  line L35 (85, 69) -> (85, -14)
  line L36 (35, 39) -> (35, 16) construction
  line L37 (66, 57) -> (66, 55)
  line L38 (70, 53) -> (70, 55)
  line L39 (66, 53) -> (66, 51)
  line L40 (68, 53) -> (70, 53)
  line L41 (64, 55) -> (64, 53)
  line L42 (64, 53) -> (66, 53)
  line L43 (68, 51) -> (68, 53)
  line L44 (70, 55) -> (68, 55)
  line L45 (66, 55) -> (64, 55)
  line L46 (66, 51) -> (68, 51)
  line L47 (68, 55) -> (68, 57)
  line L48 (66, 55) -> (64, 55)
  line L49 (68, 57) -> (66, 57)
  line L50 (70, 55) -> (68, 55)
  line L51 (66, 53) -> (66, 51)
  line L52 (66, 51) -> (68, 51)
  line L53 (68, 53) -> (70, 53)
  line L54 (64, 53) -> (66, 53)
  line L55 (64, 55) -> (64, 53)
  line L56 (70, 53) -> (70, 55)
  line L57 (68, 51) -> (68, 53)
  line L58 (66, 57) -> (66, 55)
  line L59 (68, 55) -> (68, 57)
  line L60 (68, 57) -> (66, 57)
  line L61 (32, 53) -> (32, 55)
  line L62 (36, 51) -> (34, 51)
  line L63 (36, 57) -> (36, 55)
  line L64 (36, 53) -> (36, 51)
  line L65 (34, 57) -> (36, 57)
  line L66 (34, 51) -> (34, 53)
  line L67 (38, 53) -> (36, 53)
  line L68 (36, 51) -> (34, 51)
  line L69 (36, 53) -> (36, 51)
  line L70 (36, 55) -> (38, 55)
  line L71 (36, 55) -> (38, 55)
  line L72 (38, 55) -> (38, 53)
  line L73 (36, 57) -> (36, 55)
  line L74 (32, 53) -> (32, 55)
  line L75 (34, 53) -> (32, 53)
  line L76 (34, 55) -> (34, 57)
  line L77 (34, 53) -> (32, 53)
  line L78 (38, 53) -> (36, 53)
  line L79 (38, 55) -> (38, 53)
  line L80 (32, 55) -> (34, 55)
  line L81 (34, 51) -> (34, 53)
  line L82 (34, 57) -> (36, 57)
  line L83 (32, 55) -> (34, 55)
  line L84 (34, 55) -> (34, 57)
  line L85 (4, 30) -> (4, 28)
  line L86 (34, 30) -> (36, 30)
  line L87 (34, 28) -> (34, 30)
  line L88 (6, 28) -> (6, 26)
  line L89 (6, 28) -> (6, 26)
  line L90 (38, 26) -> (36, 26)
  line L91 (38, 26) -> (36, 26)
  line L92 (4, 26) -> (4, 24)
  line L93 (68, 26) -> (70, 26)
  line L94 (66, 28) -> (64, 28)
  line L95 (2, 24) -> (2, 26)
  line L96 (4, 26) -> (4, 24)
  line L97 (70, 28) -> (68, 28)
  line L98 (66, 28) -> (64, 28)
  line L99 (2, 24) -> (2, 26)
  line L100 (2, 26) -> (0, 26)
  line L101 (38, 28) -> (38, 26)
  line L102 (34, 28) -> (34, 30)
  line L103 (36, 30) -> (36, 28)
  line L104 (36, 26) -> (36, 24)
  line L105 (32, 28) -> (34, 28)
  line L106 (34, 24) -> (34, 26)
  line L107 (38, 28) -> (38, 26)
  line L108 (36, 24) -> (34, 24)
  line L109 (32, 28) -> (34, 28)
  line L110 (66, 30) -> (66, 28)
  line L111 (68, 28) -> (68, 30)
  line L112 (68, 28) -> (68, 30)
  line L113 (32, 26) -> (32, 28)
  line L114 (34, 24) -> (34, 26)
  line L115 (34, 30) -> (36, 30)
  line L116 (36, 28) -> (38, 28)
  line L117 (34, 26) -> (32, 26)
  line L118 (66, 26) -> (66, 24)
  line L119 (4, 28) -> (6, 28)
  line L120 (66, 24) -> (68, 24)
  line L121 (64, 28) -> (64, 26)
  line L122 (70, 26) -> (70, 28)
  line L123 (4, 28) -> (6, 28)
  line L124 (2, 30) -> (4, 30)
  line L125 (66, 26) -> (66, 24)
  line L126 (2, 30) -> (4, 30)
  line L127 (70, 26) -> (70, 28)
  line L128 (68, 30) -> (66, 30)
  line L129 (68, 30) -> (66, 30)
  line L130 (6, 26) -> (4, 26)
  line L131 (4, 24) -> (2, 24)
  line L132 (6, 26) -> (4, 26)
  line L133 (66, 30) -> (66, 28)
  line L134 (4, 24) -> (2, 24)
  line L135 (36, 30) -> (36, 28)
  line L136 (36, 26) -> (36, 24)
  line L137 (32, 26) -> (32, 28)
  line L138 (34, 26) -> (32, 26)
  line L139 (36, 24) -> (34, 24)
  line L140 (36, 28) -> (38, 28)
  line L141 (4, 30) -> (4, 28)
  line L142 (68, 26) -> (70, 26)
  line L143 (64, 26) -> (66, 26)
  line L144 (64, 26) -> (66, 26)
  line L145 (0, 28) -> (2, 28)
  line L146 (2, 28) -> (2, 30)
  line L147 (0, 28) -> (2, 28)
  line L148 (0, 26) -> (0, 28)
  line L149 (70, 28) -> (68, 28)
  line L150 (66, 24) -> (68, 24)
  line L151 (68, 24) -> (68, 26)
  line L152 (64, 28) -> (64, 26)
  line L153 (2, 26) -> (0, 26)
  line L154 (2, 28) -> (2, 30)
  line L155 (0, 26) -> (0, 28)
  line L156 (68, 24) -> (68, 26)
  line L157 (4, 6) -> (4, 4)
  line L158 (34, 6) -> (36, 6)
  line L159 (34, 4) -> (34, 6)
  line L160 (6, 4) -> (6, 2)
  line L161 (6, 4) -> (6, 2)
  line L162 (38, 2) -> (36, 2)
  line L163 (38, 2) -> (36, 2)
  line L164 (4, 2) -> (4, 0)
  line L165 (68, 2) -> (70, 2)
  line L166 (66, 4) -> (64, 4)
  line L167 (2, 0) -> (2, 2)
  line L168 (4, 2) -> (4, 0)
  line L169 (70, 4) -> (68, 4)
  line L170 (66, 4) -> (64, 4)
  line L171 (2, 0) -> (2, 2)
  line L172 (2, 2) -> (0, 2)
  line L173 (38, 4) -> (38, 2)
  line L174 (34, 4) -> (34, 6)
  line L175 (36, 6) -> (36, 4)
  line L176 (36, 2) -> (36, 0)
  line L177 (32, 4) -> (34, 4)
  line L178 (34, 0) -> (34, 2)
  line L179 (38, 4) -> (38, 2)
  line L180 (36, 0) -> (34, 0)
  line L181 (32, 4) -> (34, 4)
  line L182 (66, 6) -> (66, 4)
  line L183 (68, 4) -> (68, 6)
  line L184 (68, 4) -> (68, 6)
  line L185 (32, 2) -> (32, 4)
  line L186 (34, 0) -> (34, 2)
  line L187 (34, 6) -> (36, 6)
  line L188 (36, 4) -> (38, 4)
  line L189 (34, 2) -> (32, 2)
  line L190 (66, 2) -> (66, 0)
  line L191 (4, 4) -> (6, 4)
  line L192 (66, 0) -> (68, 0)
  line L193 (64, 4) -> (64, 2)
  line L194 (70, 2) -> (70, 4)
  line L195 (4, 4) -> (6, 4)
  line L196 (2, 6) -> (4, 6)
  line L197 (66, 2) -> (66, 0)
  line L198 (2, 6) -> (4, 6)
  line L199 (70, 2) -> (70, 4)
  line L200 (68, 6) -> (66, 6)
  line L201 (68, 6) -> (66, 6)
  line L202 (6, 2) -> (4, 2)
  line L203 (4, 0) -> (2, 0)
  line L204 (6, 2) -> (4, 2)
  line L205 (66, 6) -> (66, 4)
  line L206 (4, 0) -> (2, 0)
  line L207 (36, 6) -> (36, 4)
  line L208 (36, 2) -> (36, 0)
  line L209 (32, 2) -> (32, 4)
  line L210 (34, 2) -> (32, 2)
  line L211 (36, 0) -> (34, 0)
  line L212 (36, 4) -> (38, 4)
  line L213 (4, 6) -> (4, 4)
  line L214 (68, 2) -> (70, 2)
  line L215 (64, 2) -> (66, 2)
  line L216 (64, 2) -> (66, 2)
  line L217 (0, 4) -> (2, 4)
  line L218 (2, 4) -> (2, 6)
  line L219 (0, 4) -> (2, 4)
  line L220 (0, 2) -> (0, 4)
  line L221 (70, 4) -> (68, 4)
  line L222 (66, 0) -> (68, 0)
  line L223 (68, 0) -> (68, 2)
  line L224 (64, 4) -> (64, 2)
  line L225 (2, 2) -> (0, 2)
  line L226 (2, 4) -> (2, 6)
  line L227 (0, 2) -> (0, 4)
  line L228 (68, 0) -> (68, 2)
  line L229 (135, -64) -> (-65, -64)
  line L230 (-65, -64) -> (-65, 119)
  line L231 (-65, 119) -> (135, 119)
  line L232 (135, 119) -> (135, -64)
  dimension "d199" = -30
  dimension "d206" = -80
  constraint coincident L6.start L10.start
  constraint coincident L6.end L8.start
  constraint coincident L4.start L8.end
  constraint coincident L4.end L5.start
  constraint coincident L5.end L7.end
  constraint coincident L9.end L11.end
  constraint coincident L22.end L23.end
  constraint coincident L15.start L20.start
  constraint coincident L15.end L17.start
  constraint coincident L17.end L18.start
  constraint coincident L14.start L16.start
  constraint coincident L14.end L16.end
  constraint horizontal L28
  constraint vertical L29
  constraint horizontal L30
  constraint vertical L31
  constraint coincident L2.end L3.start
  constraint coincident L0.end L1.start
  constraint midpoint L0 L36.start
  constraint midpoint L2 L36.end
  constraint symmetric L6.end L36 L44.end
  constraint symmetric L4.end L36 L37.start
  constraint symmetric L14.start L36 L40.start
  constraint symmetric L15.start L36 L39.start
  constraint symmetric L5.end L36 L37.end
  constraint symmetric L4.start L36 L47.end
  constraint symmetric L6.start L36 L38.end
  constraint symmetric L22.end L36 L41.end
  constraint symmetric L15.end L36 L39.end
  constraint symmetric L17.end L36 L43.start
  constraint symmetric L14.end L36 L38.start
  constraint symmetric L9.end L36 L41.start
  constraint coincident L61.end L74.end
  constraint coincident L76.start L80.end
  constraint coincident L65.start L76.end
  constraint coincident L63.start L65.end
  constraint coincident L63.end L70.start
  constraint coincident L70.end L71.end
  constraint coincident L67.start L72.end
  constraint coincident L64.start L67.end
  constraint coincident L62.start L64.end
  constraint coincident L62.end L66.start
  constraint coincident L66.end L75.start
  constraint coincident L61.start L74.start
  constraint coincident L145.start L147.start
  constraint coincident L145.end L146.start
  constraint coincident L124.start L126.start
  constraint coincident L85.start L124.end
  constraint coincident L85.end L119.start
  constraint coincident L88.start L89.start
  constraint coincident L88.end L89.end
  constraint coincident L92.start L96.start
  constraint coincident L92.end L96.end
  constraint coincident L95.start L99.start
  constraint coincident L95.end L99.end
  constraint coincident L100.end L148.start
  constraint coincident L105.start L109.start
  constraint coincident L87.start L102.start
  constraint coincident L86.start L87.end
  constraint coincident L86.end L103.start
  constraint coincident L103.end L116.start
  constraint coincident L101.start L107.start
  constraint coincident L90.start L91.start
  constraint coincident L90.end L91.end
  constraint coincident L104.end L108.start
  constraint coincident L106.start L108.end
  constraint coincident L106.end L114.end
  constraint coincident L113.start L117.end
  constraint coincident L217.start L219.start
  constraint coincident L217.end L218.start
  constraint coincident L196.start L198.start
  constraint coincident L157.start L196.end
  constraint coincident L157.end L191.start
  constraint coincident L160.start L161.start
  constraint coincident L160.end L161.end
  constraint coincident L164.start L168.start
  constraint coincident L164.end L168.end
  constraint coincident L167.start L171.start
  constraint coincident L167.end L171.end
  constraint coincident L172.end L220.start
  constraint coincident L177.start L181.start
  constraint coincident L159.start L174.start
  constraint coincident L158.start L159.end
  constraint coincident L158.end L175.start
  constraint coincident L175.end L188.start
  constraint coincident L173.start L179.start
  constraint coincident L162.start L163.start
  constraint coincident L162.end L163.end
  constraint coincident L176.end L180.start
  constraint coincident L178.start L180.end
  constraint coincident L178.end L186.end
  constraint coincident L185.start L189.end
extrude "拉伸41" cut 2 faces at (13.3333, -31.3333, -47) (56.6667, -31.3333, -47) along direction (0, 0, 1) blind 7 on bodies 10 bodies 10
extrude "拉伸42" add sketch "草图14" against normal blind 5 contours L4 L5 L6 L7 L8 L9 L10 L11 L12 L13 L14 L15 L16 L17 L18 L19 L20 L21 L22 L23 L24 L25 L26 L27 | L32 L33 L34 L35 | L37 L38 L39 L40 L41 L42 L43 L44 L45 L46 L47 L48 L49 L50 L51 L52 L53 L54 L55 L56 L57 L58 L59 L60 | L61 L62 L63 L64 L65 L66 L67 L68 L69 L70 L71 L72 L73 L74 L75 L76 L77 L78 L79 L80 L81 L82 L83 L84 | L85 L88 L89 L92 L95 L96 L99 L100 L119 L123 L124 L126 L130 L131 L132 L134 L141 L145 L146 L147 L148 L153 L154 L155 | L93 L94 L97 L98 L110 L111 L112 L118 L120 L121 L122 L125 L127 L128 L129 L133 L142 L143 L144 L149 L150 L151 L152 L156 | L157 L160 L161 L164 L167 L168 L171 L172 L191 L195 L196 L198 L202 L203 L204 L206 L213 L217 L218 L219 L220 L225 L226 L227 | L158 L159 L162 L163 L173 L174 L175 L176 L177 L178 L179 L180 L181 L185 L186 L187 L188 L189 L207 L208 L209 L210 L211 L212 | L165 L166 L169 L170 L182 L183 L184 L190 L192 L193 L194 L197 L199 L200 L201 L205 L214 L215 L216 L221 L222 L223 L224 L228 bodies 10
extrude "拉伸43" add sketch "草图14" along normal blind 4 contours L4 L5 L6 L7 L8 L9 L10 L11 L12 L13 L14 L15 L16 L17 L18 L19 L20 L21 L22 L23 L24 L25 L26 L27 | L37 L38 L39 L40 L41 L42 L43 L44 L45 L46 L47 L48 L49 L50 L51 L52 L53 L54 L55 L56 L57 L58 L59 L60 | L61 L62 L63 L64 L65 L66 L67 L68 L69 L70 L71 L72 L73 L74 L75 L76 L77 L78 L79 L80 L81 L82 L83 L84 | L85 L88 L89 L92 L95 L96 L99 L100 L119 L123 L124 L126 L130 L131 L132 L134 L141 L145 L146 L147 L148 L153 L154 L155 | L86 L87 L90 L91 L101 L102 L103 L104 L105 L106 L107 L108 L109 L113 L114 L115 L116 L117 L135 L136 L137 L138 L139 L140 | L93 L94 L97 L98 L110 L111 L112 L118 L120 L121 L122 L125 L127 L128 L129 L133 L142 L143 L144 L149 L150 L151 L152 L156 | L157 L160 L161 L164 L167 L168 L171 L172 L191 L195 L196 L198 L202 L203 L204 L206 L213 L217 L218 L219 L220 L225 L226 L227 | L158 L159 L162 L163 L173 L174 L175 L176 L177 L178 L179 L180 L181 L185 L186 L187 L188 L189 L207 L208 L209 L210 L211 L212 | L165 L166 L169 L170 L182 L183 L184 L190 L192 L193 L194 L197 L199 L200 L201 L205 L214 L215 L216 L221 L222 L223 L224 L228 bodies 10
extrude "拉伸44" cut 1 faces at (15, -31.3333, -61.3333) along direction (1, 0, 0) blind 5 on bodies 10 bodies 10
extrude "拉伸45" cut 1 faces at (55, -31.3333, -61.3333) along direction (-1, 0, 0) blind 5 on bodies 10 bodies 10
move_body "移动4" bodies 9 to x (1, 0, 0) y (0, 1, 0) z (0, 0, 1) at (0, 0, 3)
equation "lanunch_lenght = 150 mm" comment "发射架长度"
equation "lanunch_width = 30 mm" comment "发射架宽度"
equation "lanunch_thickness = 2 mm" comment "发射架厚度"
equation "moter_radius = 2.5 mm" comment "步性电机轴半径"
equation "moter_plane_width = 3 mm" comment "步性电机轴平面部分宽度"
equation "trigger_gap_width = 6 mm" comment "扳机卡槽宽度"
equation "trigger_radius = 20 mm" comment "扳机半径"
equation "lanunch_band_lenght = 110 mm" comment "扳机到发射架前端的距离"
equation "sevro_moter_width = 13 mm" comment "sevro马达的宽度"
equation "sevro_moter_length = 27 mm" comment "sevro马达总长度"
equation "sevro_moter_height = 17 mm" comment "sevro马达高度"
equation "d46 = lanunch_width"
equation "d47 = lanunch_band_lenght"
equation "d48 = lanunch_lenght"
equation "d49 = trigger_gap_width"
equation "d50 = trigger_radius * 2"
equation "d51 = sevro_moter_width"
equation "d52 = sevro_moter_length"
equation "cross_diameter = 6 mm" comment "十字卡槽直径"
equation "d60 = cross_diameter / 3"
equation "d61 = cross_diameter / 3"
equation "d62 = cross_diameter / 3"
equation "d63 = cross_diameter / 3"
equation "d64 = cross_diameter / 3"
equation "d65 = cross_diameter / 3"
equation "d66 = cross_diameter / 3"
equation "d67 = cross_diameter / 3"
equation "d68 = cross_diameter / 3"
equation "d69 = cross_diameter / 3"
equation "d70 = cross_diameter / 3"
equation "d71 = cross_diameter / 3"
equation "d90 = sevro_moter_length"
equation "d91 = cross_diameter / 3"
equation "d92 = cross_diameter / 3"
equation "d93 = cross_diameter / 3"
equation "d94 = cross_diameter / 3"
equation "d95 = cross_diameter / 3"
equation "d96 = cross_diameter / 3"
equation "d97 = cross_diameter / 3"
equation "d98 = cross_diameter / 3"
equation "d99 = cross_diameter / 3"
equation "d100 = cross_diameter / 3"
equation "d101 = cross_diameter / 3"
equation "d102 = cross_diameter / 3"
equation "sevro_moter_length2 = 16.5 mm" comment "sevro马达后半部分长度"
equation "sevro_moter_length3 = 3 mm" comment "sevro马达凸起部分厚度"
equation "d105 = sevro_moter_length2"
equation "d106 = sevro_moter_length3"
equation "d107 = lanunch_thickness * 1.5"
equation "fixed_object_height = 20 mm" comment "固定件2的高度"
equation "d110 = -fixed_object_height"
equation "d112 = -sevro_moter_height"
equation "d114 = -fixed_object_height"
equation "d134 = sevro_moter_width"
equation "protrusion_width = 10 mm" comment "突起处宽度"
equation "protusion_length = 5 mm" comment "突起处长度"
equation "d148 = protrusion_width"
equation "d149 = protusion_length"
equation "d152 = -sevro_moter_height"
